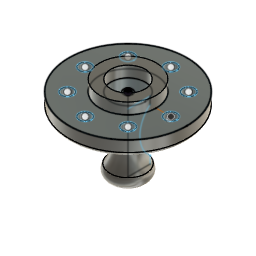
collum.switch.stand v1 (Autodesk Fusion 360 design; units mm, degrees)
Autodesk Fusion 360 part; units mm, degrees
sketch "Sketch1" plane through (0, 0, 0) normal (0, 0, 1) x (1, 0, 0)
  circle A0 centre (0, 0) radius 0.6
  circle A1 centre (0, 0) radius 8
  circle A2 centre (0, 0) radius 2.325
  circle A3 centre (0, 0) radius 3.825
  line L0 (3.825, 0.0013) -> (5.825, 0.0013) construction
  circle A4 centre (5.825, 0.0013) radius 0.8
  circle A5 centre (4.118, 4.1198) radius 0.8
  circle A6 centre (-0.0013, 5.825) radius 0.8
  circle A7 centre (-4.1198, 4.118) radius 0.8
  circle A8 centre (-5.825, -0.0013) radius 0.8
  circle A9 centre (-4.118, -4.1198) radius 0.8
  circle A10 centre (0.0013, -5.825) radius 0.8
  circle A11 centre (4.1198, -4.118) radius 0.8
  dimension "d1" = 1.2
  dimension "d2" = 16
  dimension "d3" = 4.65
  dimension "d4" = 7.65
  dimension "d5" = 2
  dimension "d6" = 1.6
  dimension "d8" = 360
  constraint coincident A0.centre A1.centre
  constraint concentric A0 A1
  constraint concentric A1 A2
  constraint concentric A2 A3
  constraint coincident A3 L0.start
  constraint horizontal L0
  constraint coincident L0.end A4.centre
  measures "d1" diameter of A0
  measures "d2" diameter of A1
  measures "d3" diameter of A2
  measures "d4" diameter of A3
  measures "d5" distance of L0.start L0.end
  measures "d6" diameter of A4
extrude "Extrude1" add sketch "Sketch1" against normal blind 2 contours A1 | A3
extrude "Extrude2" add sketch "Sketch1" along normal blind 1.5 contours A3
sketch "Sketch2" plane through (0, 0, 0) normal (1, 0, 0) x (0, 1, 0)
  line L0 (0, 0) -> (0, -10)
  line L1 (0, -10) -> (3, -10)
  line L2 (0, -2) -> (3, -2)
  line L3 (3, -10) -> (3, -9)
  line L4 (3, -2) -> (3, -3)
  arc A0 (3, -3) -> (3, -9) centre (5.5787, -6) ccw
  dimension "d13" = 10
  dimension "d14" = 3
  dimension "d24" = 1
  dimension "d25" = 1
  constraint coincident L0.start origin
  constraint vertical L0
  constraint perpendicular L0 L1
  constraint coincident L0 L2.start
  constraint perpendicular L0 L2
  constraint perpendicular L1 L3
  constraint perpendicular L2 L4
  measures "d13" distance of L0.start L0.end
  measures "d14" distance of L2.start L2.end
  measures "d24" distance of L1.end L3.end
  measures "d25" distance of L2.end L4.end
revolve "Revolve2" add sketch "Sketch2" angle 360 about axis through (0, 0, 1.75) along (0, 0, 1)
fillet "Fillet4" radius 2 1 edges at (-2.797, 1.0848, -9)
fillet "Fillet5" radius 2 1 edges at (-2.797, 1.0848, -3)
fillet "Fillet6" radius 1 1 edges at (-2.797, 1.0848, -10)
extrude "Extrude3" cut sketch "Sketch1" against normal blind 11 contours A0
fillet "Fillet8" radius 1 1 edges at (1.0848, -2.797, -2)
fillet "Fillet9" radius 0.5 1 edges at (-7.4586, 2.8929, -2)
revolve "Revolve1" [suppressed]
fillet "Fillet1" [suppressed]
fillet "Fillet2" [suppressed]
fillet "Fillet3" [suppressed]
